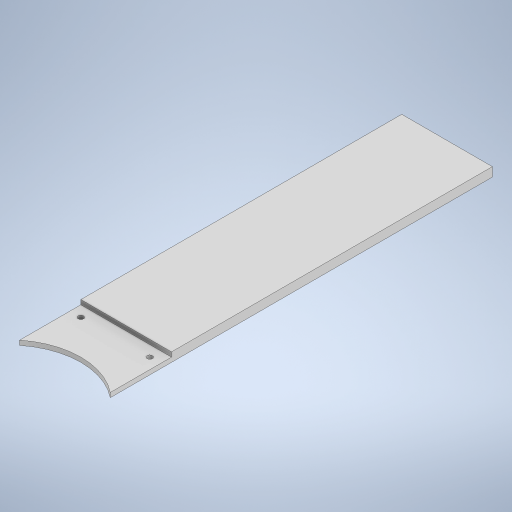
# Autodesk Inventor part: peca2_suporte
Saved by Autodesk Inventor 2024.3 (Build 283343000, 343)
## iProperties
Created: 2024-12-04
Part Number: peca2_suporte
Material: Genérico
Document SubType Name: Modeling
Designer: lostv
Density: 1 g/cm^3
Appearance: Padrão
Author: lostv
Autodesk Inventor part; units mm, degrees
ref_plane "YZ Plane" through (0, 0, 0) normal (1, 0, 0) x (0, 1, 0)
ref_plane "XZ Plane" through (0, 0, 0) normal (0, 1, 0) x (-1, 0, 0)
ref_plane "XY Plane" through (0, 0, 0) normal (0, 0, 1) x (1, 0, 0)
sketch "Esboço1" plane through (0, 0, 0) normal (0, 1, 0) x (-1, 0, 0)
  line L0 (-1.3226, 64.6966) -> (-1.3226, 176.6966) construction
  line L1 (-1.3226, 64.6966) -> (-1.3226, 179.6966) construction
  line L2 (23.6774, 24.6966) -> (-26.3226, 24.6966)
  line L3 (-26.3226, 24.6966) -> (-26.3226, -57.3034)
  line L4 (-26.3226, -57.3034) -> (23.6774, -57.3034)
  line L5 (23.6774, -57.3034) -> (23.6774, 24.6966)
  line L6 (23.6774, -57.3034) -> (-26.3226, -57.3034)
  line L7 (-26.3226, -57.3034) -> (-26.3226, -177.3034)
  line L8 (-26.3226, -177.3034) -> (23.6774, -177.3034)
  line L9 (23.6774, -177.3034) -> (23.6774, -57.3034)
  line L10 (23.6774, 24.6966) -> (23.6774, 33.4716)
  line L11 (-26.3226, 24.6966) -> (-26.3226, 33.4716)
  line L12 (23.6774, 24.6966) -> (-26.3226, 24.6966)
  line L13 (-26.3226, 24.6966) -> (-26.3226, -0.3034)
  line L14 (-26.3226, -0.3034) -> (23.6774, -0.3034)
  line L15 (23.6774, -0.3034) -> (23.6774, 24.6966)
  circle A0 centre (17.6774, 5.6966) radius 1.5
  circle A1 centre (17.6774, 5.6966) radius 2.75
  circle A2 centre (-20.3226, 5.6966) radius 1.5
  circle A3 centre (-20.3226, 5.6966) radius 2.75
  arc A4 (-26.3226, 33.4716) -> (23.6774, 33.4716) centre (-1.3226, 64.6966) ccw
  point P0 (0, 0)
  point P1 (-26.3226, -57.3034)
  dimension "d8" = 120
  dimension "d9" = 50
  dimension "d10" = 25
  dimension "d11" = 25
  dimension "d12" = 50
  dimension "d13" = 3
  dimension "d14" = 6
  dimension "d15" = 6
  dimension "d16" = 5.5
  constraints: 32 end point, 7 parallel, 5 centre point, 3 coincident, 3 horizontal, 3 perpendicular, 2 point on circle, 2 vertical, 1 point on line, 1 tangent
  measures "d8" distance of L9.start L5.start
  measures "d9" distance between parallel lines of L7 L9
  measures "d10" distance between parallel lines of L5 L1
  measures "d11" distance between parallel lines of L14 L2
  measures "d12" distance of L13.end L15.start
  measures "d13" diameter of A0
  measures "d14" distance from line of L15 A0.centre
  measures "d15" distance from line of L14 A0.centre
  measures "d16" diameter of A1
extrude "Extrusão1" add sketch "Esboço1" along normal blind 2.5 contours L5 L14 L3 L2 | L2 A4 L10 | L2 L11 A4 | A1 | A3
extrude "Extrusão2" add sketch "Esboço1" along normal blind 5 contours L5 L4 L3 L14 | L9 L8 L7 L4
